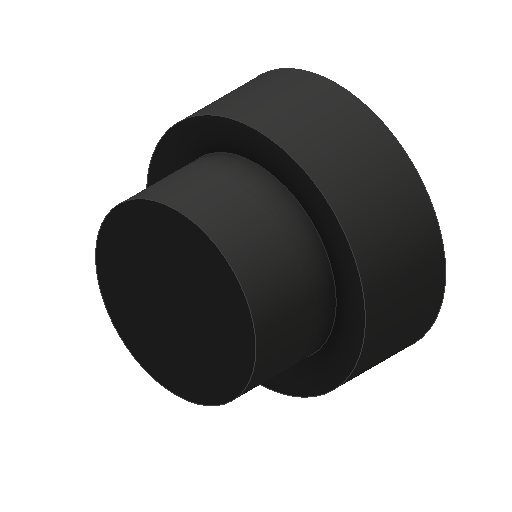
# Autodesk Inventor part: COTS_GENERIC_22mm_Industrial_Button_Green_Pause_Reset
Saved by Autodesk Inventor 2026.1 (Build 301233000, 233)
## iProperties
Created: 2016-07-19
Part Number: COTS_GENERIC_22mm_Industrial_Button_Green_Pause_Reset
Material: Ogólny
Document SubType Name: Modeling
Designer: Andrzej
Density: 1 g/cm^3
Appearance: Kauczuk — czarny
Author: Andrzej
Autodesk Inventor part; units mm, degrees
ref_plane "YZ Plane" through (0, 0, 0) normal (1, 0, 0) x (0, 1, 0)
ref_plane "XZ Plane" through (0, 0, 0) normal (0, 1, 0) x (-1, 0, 0)
ref_plane "XY Plane" through (0, 0, 0) normal (0, 0, 1) x (1, 0, 0)
sketch "Szkic1" plane through (0, 0, 0) normal (0, 0, 1) x (1, 0, 0)
  line L0 (0, 4) -> (15, 4)
  line L1 (15, 4) -> (15, -7)
  line L2 (15, -7) -> (11, -7)
  line L3 (11, -7) -> (11, -18)
  line L4 (11, -18) -> (0, -18)
  line L5 (0, -18) -> (0, 4)
  line L6 (0, -22.4) -> (0, 8.4) projected
  point P0 (0, 0)
  dimension "d0" = 15
  dimension "d1" = 11
  dimension "d2" = 4
  dimension "d3" = 11
  constraints: 12 end point, 5 perpendicular, 1 horizontal
  measures "d0" distance of L0.start L0.end
  measures "d1" distance of L0.end L1.end
  measures "d2" distance of L1.end L2.end
  measures "d3" distance of L2.end L3.end
revolve "Obrót1" add sketch "Szkic1" angle 360 about axis through (0, -10, 0) along (0, 1, 0)
sketch "Szkic2" plane through (0, 4, 0) normal (0, 1, 0) x (1, 0, 0)
  circle A0 centre (0, 0) radius 15 projected
  circle A1 centre (0, 0) radius 13
  dimension "d5" = 2
  constraints: 1 centre point
  measures "d5" radial gap between concentric circles of A0 A1
extrude "Wyciągnięcie proste1" cut sketch "Szkic2" against normal blind 0.1 contours A1
